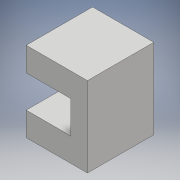
# Autodesk Inventor part: slot
Saved by Autodesk Inventor 2017.3 (Build 213256000, 256)
## iProperties
Created: 2018-06-04
Part Number: slot
Material: Generic
Document SubType Name: Modeling
Designer: JetPack Jord
Density: 1 g/cm^3
Appearance: Default
Author: JetPack Jord
Autodesk Inventor part; units mm, degrees
ref_plane "YZ Plane" through (0, 0, 0) normal (1, 0, 0) x (0, 1, 0)
ref_plane "XZ Plane" through (0, 0, 0) normal (0, 1, 0) x (-1, 0, 0)
ref_plane "XY Plane" through (0, 0, 0) normal (0, 0, 1) x (1, 0, 0)
sketch "Sketch1" plane through (0, 0, 0) normal (0, 1, 0) x (-1, 0, 0)
  line L0 (-9.2268, 12.0612) -> (9.2268, 12.0612)
  line L1 (9.2268, -12.0612) -> (-9.2268, -12.0612)
  line L2 (-9.2268, -12.0612) -> (-9.2268, 12.0612)
  line L3 (-9.2268, 12.0612) -> (9.2268, -12.0612) construction
  line L4 (9.2268, 12.0612) -> (-9.2268, -12.0612) construction
  line L5 (-4.2415, 4.8647) -> (9.2268, 4.8647)
  line L6 (9.2268, -4.8647) -> (-4.2415, -4.8647)
  line L7 (-4.2415, -4.8647) -> (-4.2415, 4.8647)
  line L8 (-4.2415, 4.8647) -> (14.8956, -4.8647) construction
  line L9 (14.8956, 4.8647) -> (-4.2415, -4.8647) construction
  line L10 (9.2268, 12.0612) -> (9.2268, 4.8647)
  line L11 (9.2268, -4.8647) -> (9.2268, -12.0612)
  point P0 (0, 0)
  point P1 (5.327, 0)
  constraints: 24 end point, 4 midpoint, 4 parallel, 2 horizontal, 2 perpendicular
extrude "Extrusion1" add sketch "Sketch1" along normal blind 20
body "Solid1"
